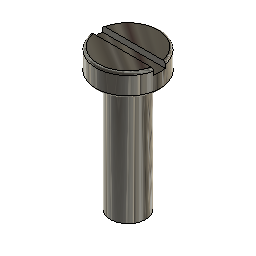
STR (Autodesk Fusion 360 archive; units mm, degrees)
design "Tornillo M3 10mm"
Autodesk Fusion 360 part; units mm, degrees
sketch "Sketch1" plane through (0, 0, 0) normal (0, 0, 1) x (1, 0, 0) in component "Component"
  circle A0 centre (0, 0) radius 1.5
  dimension "d1" = 3
  constraint coincident A0.centre origin
  measures "d1" diameter of A0
extrude "Extrude1" add sketch "Sketch1" along normal blind 10 in component "Component"
sketch "Sketch2" plane through (0, 0, 10) normal (0, 0, 1) x (-1, 0, 0) in component "Component"
  circle A0 centre (0, 0) radius 1.5
  circle A1 centre (0, 0) radius 2.7
  dimension "d8" = 5.4
  constraint coincident A0.centre A1.centre
  measures "d8" diameter of A1
extrude "Extrude2" add sketch "Sketch2" along normal blind 1.9 contours A0 | A1 in component "Component"
fillet "Fillet2" radius 0.2 2 edges at (2.5173, 0.9764, 11.9) (2.5173, 0.9764, 10) in component "Component"
sketch "Sketch3" plane through (0, 0, 11.9) normal (0, 0, 1) x (-1, 0, 0) in component "Component"
  circle A0 centre (0, 0) radius 2.5
  line L0 (-2.7, 0.5) -> (2.7, 0.5)
  line L1 (2.7, 0.5) -> (2.7, -0.5)
  line L2 (2.7, -0.5) -> (-2.7, -0.5)
  line L3 (-2.7, -0.5) -> (-2.7, 0.5)
  line L4 (-2.7, 0.5) -> (2.7, -0.5) construction
  line L5 (2.7, 0.5) -> (-2.7, -0.5) construction
  dimension "d10" = 5.4
  dimension "d11" = 1
  constraint horizontal L0
  constraint perpendicular L0 L1
  constraint parallel L0 L2
  constraint parallel L1 L3
  constraint coincident L4 A0.centre
  constraint coincident L5 A0.centre
  constraint coincident A0.centre origin
  measures "d10" distance of L1.end L2.end
  measures "d11" distance of L0.end L1.end
extrude "Extrude3" cut sketch "Sketch3" against normal blind 0.5 contours A0 L0 L2 | A0 L0 L1 L2 | A0 L0 L2 L3 in component "Component"
component "Tornillo M3 10mm v2 (1)" placed x (1, 0, 0) y (0, 1, 0) z (0, 0, 1) at (0, 0, 0)
component "Component" placed x (1, 0, 0) y (0, 1, 0) z (0, 0, 1) at (0, 0, 0) in component "Tornillo M3 10mm v2 (1)"
